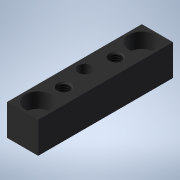
# Autodesk Inventor part: 722627 MUE-70/80P2
Saved by Autodesk Inventor 2021 (Build 250183000, 183)
## iProperties
Created: 2026-04-18
Part Number: 722627 MUE-70/80P2
Material: Generic
Catalog Web Link: www.3dfindit.com
Description: MUE-P2-terminal strip
Vendor: FESTO
Document SubType Name: Modeling
Designer: psAdmin
Manufacturer: FESTO
Mass: 5.71937 g
Surface Area: 36.6268 cm^2
Volume: 5.71937 cm^3
Density: 1 g/cm^3
Appearance: PSOLRGB-176-176-176
Category: PARTsolutions
Company: FESTO
Title: 722627 MUE-70/80P2
Author: Cadenas PARTsolutions
Comments: terminal strip
PSOL_IDENT_0: {$CADENAS_DATA/23d-libs/festo/parts/m/mue/parts/mue_2.prj},176 {VTYP=3D},{NB=722627 MUE-70/80P2},{LI
PSOL_IDENT_1: NA=722627 MUE-70/80P2},{NN=MUE-P2},{DATE=30.06.2025 07:27:24},{GEOMDATE=16.01.2017 12:17:00},{VERSIO
PSOL_IDENT_2: N=},{LINEID=20},{WBVAR=},{WBNUMERIC=}  {NB=722627 MUE-70/80P2},{LINA=722627 MUE-70/80P2},{KT=DUMMY},
PSOL_IDENT_3: {TNR=722627},{TYP=MUE-70/80},{V=3},{B=12.000},{B1=52.000},{B2=12.000},{H=40.000}
NB: 722627 MUE-70/80P2
NN: MUE-P2
NT: terminal strip
NBSYN: $TNR. $TYP.P2
LINA: 722627 MUE-70/80P2
CATALOG: Festo
TNR: 722627
TYP: MUE-70/80
V: 3
B: 12
B1: 52
B2: 12
H: 40
SUPPLIER: FESTO
ARTICLENO: 722627 MUE-70/80P2
BOMINFO: 722627 MUE-70/80P2
CREATOR: CADENAS GmbH
Autodesk Inventor part; units mm, degrees
sketch "Sketch_4" plane through (0, 0, 0) normal (0, 0, 1) x (1, 0, 0)
  line L0 (-6, 12) -> (-6, 0)
  line L1 (-6, 0) -> (6, 0)
  line L2 (6, 0) -> (6, 12)
  line L3 (6, 12) -> (-6, 12)
  constraints: 8 end point
extrude "Extrusion1" add sketch "Sketch_4" along normal mid plane 52
sketch "Sketch2" plane through (-6, 12, 26) normal (0, 1, 0) x (1, 0, 0)
  point P0 (6, 46)
hole "Hole1" at (0, 12, -20) direction (0, -1, 0) diameter 5.5 depth 12 counterbore diameter 10 counterbore depth 5.8
sketch "Sketch3" plane through (-6, 12, 26) normal (0, 1, 0) x (1, 0, 0)
  point P0 (6, 6)
hole "Hole2" at (0, 12, 20) direction (0, -1, 0) diameter 5.5 depth 12 counterbore diameter 10 counterbore depth 5.8
sketch "Sketch_13" plane through (0, 0, 0) normal (1, 0, 0) x (0, 0, -1)
  line L0 (10, 0) -> (10, 12)
  line L1 (10, 12) -> (12.5, 12)
  line L2 (12.5, 12) -> (12.067, 11.567)
  line L3 (12.067, 11.567) -> (12.067, 0.433)
  line L4 (12.067, 0.433) -> (12.5, 0)
  line L5 (12.5, 0) -> (10, 0)
  line L6 (10, 0) -> (10, 12)
  constraints: 14 end point
revolve "Revolution1" cut sketch "Sketch_13" angle 360 about axis through (0, 0, -10) along (0, -1, 0)
thread "Thread1" size "M5x0.8" class "6H" standard "ISO Metric profile" full length
sketch "Sketch_14" plane through (0, 0, 0) normal (1, 0, 0) x (0, 0, -1)
  line L0 (-10, 0) -> (-10, 12)
  line L1 (-10, 12) -> (-7.5, 12)
  line L2 (-7.5, 12) -> (-7.933, 11.567)
  line L3 (-7.933, 11.567) -> (-7.933, 0.433)
  line L4 (-7.933, 0.433) -> (-7.5, 0)
  line L5 (-7.5, 0) -> (-10, 0)
  line L6 (-10, 0) -> (-10, 12)
  constraints: 14 end point
revolve "Revolution2" cut sketch "Sketch_14" angle 360 about axis through (0, 0, 10) along (0, -1, 0)
thread "Thread2" size "M5x0.8" class "6H" standard "ISO Metric profile" full length
sketch "Sketch6" plane through (-6, 0, 26) normal (0, -1, 0) x (1, 0, 0)
  point P0 (4, -26)
hole "Hole3" at (-2, 0, 0) direction (0, 1, 0) diameter 5 depth 12
ref_plane "HGO_ANBAU_XY" through (0, 0, 0) normal (0, 1, 0) x (1, 0, 0)
ref_plane "HGO_ANBAU_YZ" through (0, 0, 0) normal (1, 0, 0) x (0, 0, -1)
ref_plane "HGO_ANBAU_ZX" through (0, 0, 0) normal (0, 0, -1) x (0, 1, 0)
ref_plane "HGO_ANBAU_Schrauben_1_XY" through (0, 5.5, -20) normal (0, -1, 0) x (1, 0, 0)
ref_plane "HGO_ANBAU_Schrauben_1_YZ" through (0, 5.5, -20) normal (1, 0, 0) x (0, 0, 1)
ref_plane "HGO_ANBAU_Schrauben_1_ZX" through (0, 5.5, -20) normal (0, 0, 1) x (0, -1, 0)
ref_plane "HGO_ANBAU_Schrauben_2_XY" through (0, 5.5, 20) normal (0, -1, 0) x (1, 0, 0)
ref_plane "HGO_ANBAU_Schrauben_2_YZ" through (0, 5.5, 20) normal (1, 0, 0) x (0, 0, 1)
ref_plane "HGO_ANBAU_Schrauben_2_ZX" through (0, 5.5, 20) normal (0, 0, 1) x (0, -1, 0)
ref_plane "KLEMMHALTER_XY" through (0, 12, 0) normal (0, 1, 0) x (1, 0, 0)
ref_plane "KLEMMHALTER_YZ" through (0, 12, 0) normal (1, 0, 0) x (0, 0, -1)
ref_plane "KLEMMHALTER_ZX" through (0, 12, 0) normal (0, 0, -1) x (0, 1, 0)
body "Solid1"
